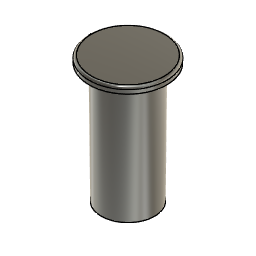
RadioGlobe-Bushing-Top v6 (Autodesk Fusion 360 design; units mm, degrees)
Autodesk Fusion 360 part; units mm, degrees
note: some values were not read from the file. Set by a fixed rule: which sketch regions a step uses.
sketch "Sketch11" plane through (0, 0, 0) normal (0, 0, 1) x (1, 0, 0)
  line L0 (-5.5, 75.0001) -> (0, 75)
  line L1 (0, 101) -> (0, 75)
  line L2 (-5.5, 75.0001) -> (-5.7349, 99.8354)
  arc A0 (-5.7349, 99.8354) -> (-8, 99.6795) centre (0, 0) ccw
  line L3 (-8, 99.6795) -> (-8, 101.0839)
  line L4 (-8, 101) -> (0, 101)
  dimension "d25" = 200
  dimension "d27" = 5.5
  constraint coincident A0.centre origin
  constraint vertical L3
  constraint coincident L3 L4.start
  constraint perpendicular L1 L4
  measures "d25" diameter of A0
  measures "d27" distance of L0.end L0.start
revolve "Revolve3" add sketch "Sketch11" angle 360 about axis through (0, 101, 0) along (0, -1, 0)
sketch "Sketch12" plane through (0, 85, 0) normal (0, -1, 0) x (1, 0, 0)
  circle A0 centre (0, 0) radius 4
  circle A1 centre (0, 0) radius 2.1
  circle A2 centre (0, 0) radius 5.5
  dimension "d29" = 4.2
  constraint coincident A0.centre A1.centre
  measures "d29" diameter of A1
extrude "Extrude4" cut sketch "Sketch12" along normal blind -10 and the other way blind -11 contours A1
move_body "Move1" bodies 1 to x (1, 0, 0) y (0, 0, 1) z (0, -1, 0) at (0, 80, -80)
fillet "Fillet3" radius 0.5 tangency weight 0.84007 1 edges at (-7.4586, 77.1071, 21)
